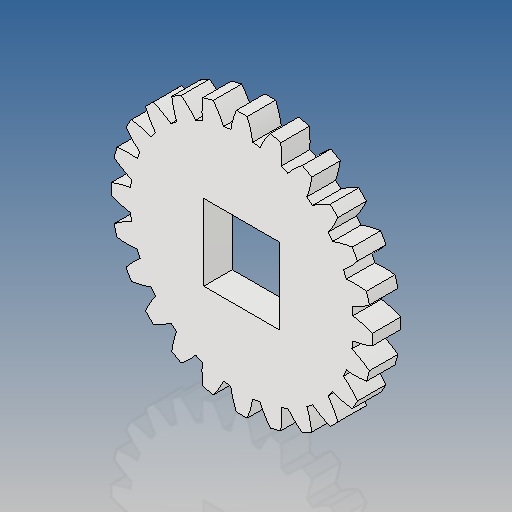
# Autodesk Inventor part: engrane motor-dado
Saved by Autodesk Inventor 2017 (Build 210142000, 142)
## iProperties
Part Number: engrane motor-dado
Material: Genérico
Document SubType Name: Modeling
Designer: FABLAB
Density: 1 g/cm^3
Appearance: Blanco
Author: FABLAB
Autodesk Inventor part; units mm, degrees
ref_plane "YZ Plane" through (0, 0, 0) normal (1, 0, 0) x (0, 1, 0)
ref_plane "XZ Plane" through (0, 0, 0) normal (0, 1, 0) x (-1, 0, 0)
ref_plane "XY Plane" through (0, 0, 0) normal (0, 0, 1) x (1, 0, 0)
sketch "Boceto1" plane through (0, 0, 0) normal (0, 0, 1) x (1, 0, 0)
  line L0 (8, -8) -> (-8, -8) projected
  line L1 (-8, -8) -> (-8, 8) projected
  line L2 (-8, 8) -> (8, 8) projected
  line L3 (8, 8) -> (8, -8) projected
  circle A0 centre (0, 0) radius 15 construction
  circle A1 centre (0, 0) radius 27.5
  dimension "d0" = 55
  constraints: 1 centre point, 1 coincident
  measures "d0" diameter of A1
extrude "Extrusión1" add sketch "Boceto1" along normal blind 6
spur gear teeth "iFeature1:1" teeth 24 pitch diameter 48 tip diameter 56 root diameter 47 face width 7 trims to tip circle yes start plane through (0, 0, 6) normal (0, 0, 1) x (1, 0, 0)
